Autodesk Fusion 360 part; units mm, degrees
note: some values were not read from the file. Set by a fixed rule: which sketch regions a step uses.
(part 6 of 10)
  spline S32 degree 5 poles (0.6796, -14.5069) (0.6796, -14.507) (0.6797, -14.5072) (0.6797, -14.5074) (0.6797, -14.5078) (0.6797, -14.5083) (0.6798, -14.5089) (0.6798, -14.5096) (0.6799, -14.5104) (0.6799, -14.5112) (0.68, -14.5122) (0.6801, -14.5132) (0.6802, -14.5143) (0.6803, -14.5154) (0.6804, -14.5167) (0.6805, -14.518) (0.6806, -14.5193) (0.6807, -14.5208) (0.6809, -14.5223) (0.681, -14.5239) (0.6812, -14.5256) (0.6814, -14.5273) (0.6815, -14.5291) (0.6817, -14.531) (0.6819, -14.5329) (0.6822, -14.5349) (0.6824, -14.537) (0.6826, -14.5392) (0.6829, -14.5414) (0.6832, -14.5436) (0.6834, -14.546) (0.6837, -14.5484) (0.684, -14.5508) (0.6844, -14.5533) (0.6847, -14.5559) (0.685, -14.5586) (0.6854, -14.5613) (0.6858, -14.5641) (0.6862, -14.5669) (0.6866, -14.5698) (0.687, -14.5727) (0.6874, -14.5757) (0.6879, -14.5788) (0.6883, -14.5819) (0.6888, -14.5851) (0.6893, -14.5883) (0.6898, -14.5916) (0.6904, -14.595) (0.6909, -14.5984) (0.6915, -14.6018) (0.6921, -14.6054) (0.6926, -14.6089) (0.6933, -14.6125) (0.6939, -14.6162) (0.6945, -14.6199) (0.6952, -14.6237) (0.6959, -14.6275) (0.6966, -14.6314) (0.6973, -14.6354) (0.698, -14.6394) (0.6988, -14.6434) (0.6995, -14.6475) (0.7003, -14.6516) (0.7011, -14.6558) (0.702, -14.66) (0.7028, -14.6643) (0.7037, -14.6686) (0.7045, -14.673) (0.7054, -14.6774) (0.7064, -14.6819) (0.7073, -14.6864) (0.7082, -14.691) (0.7092, -14.6956) (0.7102, -14.7003) (0.7112, -14.705) (0.7123, -14.7097) (0.7133, -14.7145) (0.7144, -14.7194) (0.7155, -14.7243) (0.7166, -14.7292) (0.7177, -14.7342) (0.7189, -14.7392) (0.7201, -14.7442) (0.7213, -14.7493) (0.7225, -14.7545) (0.7237, -14.7597) (0.725, -14.7649) (0.7263, -14.7702) (0.7276, -14.7755) (0.7289, -14.7808) (0.7302, -14.7862) (0.7316, -14.7917) (0.733, -14.7971) (0.7344, -14.8027) (0.7358, -14.8082) (0.7372, -14.8138) (0.7387, -14.8194) (0.7402, -14.8251) (0.7417, -14.8308) (0.7433, -14.8366) (0.7448, -14.8424) (0.7464, -14.8482) (0.748, -14.854) (0.7496, -14.86) (0.7513, -14.8659) (0.7529, -14.8719) (0.7546, -14.8779) (0.7564, -14.8839) (0.7581, -14.89) (0.7599, -14.8961) (0.7616, -14.9023) (0.7634, -14.9085) (0.7653, -14.9147) (0.7671, -14.921) (0.769, -14.9273) (0.7709, -14.9336) (0.7728, -14.94) (0.7748, -14.9464) (0.7767, -14.9528) (0.7787, -14.9593) (0.7807, -14.9658) (0.7828, -14.9723) (0.7848, -14.9789) (0.7869, -14.9855) (0.789, -14.9921) (0.7912, -14.9987) (0.7933, -15.0054) (0.7955, -15.0122) (0.7977, -15.0189) (0.8, -15.0257) (0.8022, -15.0325) (0.8045, -15.0394) (0.8068, -15.0463) (0.8091, -15.0532) (0.8115, -15.0601) (0.8138, -15.0671) (0.8162, -15.0741) (0.8187, -15.0812) (0.8211, -15.0882) (0.8236, -15.0953) (0.8261, -15.1025) (0.8286, -15.1096) (0.8311, -15.1168) (0.8337, -15.124) (0.8363, -15.1313) (0.8389, -15.1385) (0.8416, -15.1458) (0.8442, -15.1531) (0.8469, -15.1605) (0.8497, -15.1679) (0.8524, -15.1753) (0.8552, -15.1827) (0.858, -15.1902) (0.8608, -15.1977) (0.8636, -15.2052) (0.8665, -15.2127) (0.8694, -15.2203) (0.8723, -15.2279) (0.8753, -15.2355) (0.8782, -15.2432) (0.8812, -15.2509) (0.8843, -15.2586) (0.8873, -15.2663) (0.8904, -15.274) (0.8935, -15.2818) (0.8966, -15.2896) (0.8998, -15.2974) (0.9029, -15.3053) (0.9061, -15.3132) (0.9094, -15.3211) (0.9126, -15.329) (0.9159, -15.3369) (0.9192, -15.3449) (0.9225, -15.3529) (0.9259, -15.3609) (0.9293, -15.369) (0.9327, -15.377) (0.9361, -15.3851) (0.9396, -15.3932) (0.9431, -15.4014) (0.9466, -15.4095) (0.9501, -15.4177) (0.9537, -15.4259) (0.9573, -15.4341) (0.9609, -15.4424) (0.9646, -15.4507) (0.9682, -15.459) (0.9719, -15.4673) (0.9757, -15.4756) (0.9794, -15.484) (0.9832, -15.4923) (0.987, -15.5007) (0.9908, -15.5091) (0.9947, -15.5176) (0.9986, -15.526) (1.0025, -15.5345) (1.0064, -15.543) (1.0104, -15.5515) (1.0144, -15.5601) (1.0184, -15.5686) (1.0224, -15.5772) (1.0265, -15.5858) (1.0306, -15.5944) (1.0347, -15.6031) (1.0389, -15.6117) (1.043, -15.6204) (1.0472, -15.6291) (1.0515, -15.6378) (1.0557, -15.6466) (1.06, -15.6553) (1.0643, -15.6641) (1.0687, -15.6729) (1.073, -15.6817) (1.0774, -15.6905) (1.0818, -15.6993) (1.0863, -15.7082) (1.0907, -15.7171) (1.0952, -15.726) (1.0998, -15.7349) (1.1043, -15.7438) (1.1089, -15.7528) (1.1135, -15.7617) (1.1182, -15.7707) (1.1228, -15.7797) (1.1275, -15.7887) (1.1322, -15.7977) (1.137, -15.8068) (1.1417, -15.8159) (1.1465, -15.8249) (1.1514, -15.834) (1.1562, -15.8431) (1.1611, -15.8523) (1.166, -15.8614) (1.1709, -15.8706) (1.1759, -15.8797) (1.1809, -15.8889) (1.1859, -15.8981) (1.1909, -15.9074) (1.196, -15.9166) (1.2011, -15.9258) (1.2062, -15.9351) (1.2104, -15.9425) (1.2135, -15.9481) (1.2155, -15.9518) (1.2166, -15.9537) knots 0 0 0 0 0 0 0.00416667 0.00833333 0.0125 0.01666667 0.02083333 0.025 0.02916667 0.03333333 0.0375 0.04166667 0.04583333 0.05 0.05416667 0.05833333 0.0625 0.06666667 0.07083333 0.075 0.07916667 0.08333333 0.0875 0.09166667 0.09583333 0.1 0.10416667 0.10833333 0.1125 0.11666667 0.12083333 0.125 0.12916667 0.13333333 0.1375 0.14166667 0.14583333 0.15 0.15416667 0.15833333 0.1625 0.16666667 0.17083333 0.175 0.17916667 0.18333333 0.1875 0.19166667 0.19583333 0.2 0.20416667 0.20833333 0.2125 0.21666667 0.22083333 0.225 0.22916667 0.23333333 0.2375 0.24166667 0.24583333 0.25 0.25416667 0.25833333 0.2625 0.26666667 0.27083333 0.275 0.27916667 0.28333333 0.2875 0.29166667 0.29583333 0.3 0.30416667 0.30833333 0.3125 0.31666667 0.32083333 0.325 0.32916667 0.33333333 0.3375 0.34166667 0.34583333 0.35 0.35416667 0.35833333 0.3625 0.36666667 0.37083333 0.375 0.37916667 0.38333333 0.3875 0.39166667 0.39583333 0.4 0.40416667 0.40833333 0.4125 0.41666667 0.42083333 0.425 0.42916667 0.43333333 0.4375 0.44166667 0.44583333 0.45 0.45416667 0.45833333 0.4625 0.46666667 0.47083333 0.475 0.47916667 0.48333333 0.4875 0.49166667 0.49583333 0.5 0.50416667 0.50833333 0.5125 0.51666667 0.52083333 0.525 0.52916667 0.53333333 0.5375 0.54166667 0.54583333 0.55 0.55416667 0.55833333 0.5625 0.56666667 0.57083333 0.575 0.57916667 0.58333333 0.5875 0.59166667 0.59583333 0.6 0.60416667 0.60833333 0.6125 0.61666667 0.62083333 0.625 0.62916667 0.63333333 0.6375 0.64166667 0.64583333 0.65 0.65416667 0.65833333 0.6625 0.66666667 0.67083333 0.675 0.67916667 0.68333333 0.6875 0.69166667 0.69583333 0.7 0.70416667 0.70833333 0.7125 0.71666667 0.72083333 0.725 0.72916667 0.73333333 0.7375 0.74166667 0.74583333 0.75 0.75416667 0.75833333 0.7625 0.76666667 0.77083333 0.775 0.77916667 0.78333333 0.7875 0.79166667 0.79583333 0.8 0.80416667 0.80833333 0.8125 0.81666667 0.82083333 0.825 0.82916667 0.83333333 0.8375 0.84166667 0.84583333 0.85 0.85416667 0.85833333 0.8625 0.86666667 0.87083333 0.875 0.87916667 0.88333333 0.8875 0.89166667 0.89583333 0.9 0.90416667 0.90833333 0.9125 0.91666667 0.92083333 0.925 0.92916667 0.93333333 0.9375 0.94166667 0.94583333 0.95 0.95416667 0.95833333 0.9625 0.96666667 0.97083333 0.975 0.97916667 0.98333333 0.9875 0.99166667 0.99583333 1 1 1 1 1 1
  arc A41 (4.5069, -15.3521) -> (5.3776, -15.0692) centre (0, 0) ccw
  spline S33 degree 5 poles (-15.5488, -3.7729) (-15.5467, -3.7733) (-15.5425, -3.7742) (-15.5363, -3.7754) (-15.5279, -3.777) (-15.5175, -3.779) (-15.5072, -3.781) (-15.4968, -3.783) (-15.4865, -3.7849) (-15.4762, -3.7869) (-15.4659, -3.7888) (-15.4556, -3.7907) (-15.4454, -3.7925) (-15.4352, -3.7944) (-15.425, -3.7962) (-15.4148, -3.798) (-15.4047, -3.7998) (-15.3946, -3.8015) (-15.3845, -3.8033) (-15.3744, -3.805) (-15.3644, -3.8067) (-15.3544, -3.8083) (-15.3444, -3.81) (-15.3344, -3.8116) (-15.3244, -3.8132) (-15.3145, -3.8148) (-15.3046, -3.8164) (-15.2947, -3.8179) (-15.2849, -3.8195) (-15.2751, -3.821) (-15.2653, -3.8225) (-15.2555, -3.8239) (-15.2457, -3.8254) (-15.236, -3.8268) (-15.2263, -3.8282) (-15.2166, -3.8296) (-15.207, -3.831) (-15.1974, -3.8323) (-15.1878, -3.8337) (-15.1782, -3.835) (-15.1687, -3.8363) (-15.1591, -3.8375) (-15.1497, -3.8388) (-15.1402, -3.84) (-15.1308, -3.8412) (-15.1214, -3.8424) (-15.112, -3.8436) (-15.1026, -3.8448) (-15.0933, -3.8459) (-15.084, -3.847) (-15.0747, -3.8481) (-15.0655, -3.8492) (-15.0563, -3.8503) (-15.0471, -3.8513) (-15.0379, -3.8523) (-15.0288, -3.8533) (-15.0197, -3.8543) (-15.0106, -3.8553) (-15.0015, -3.8562) (-14.9925, -3.8572) (-14.9835, -3.8581) (-14.9746, -3.859) (-14.9656, -3.8598) (-14.9567, -3.8607) (-14.9479, -3.8615) (-14.939, -3.8624) (-14.9302, -3.8632) (-14.9214, -3.8639) (-14.9127, -3.8647) (-14.9039, -3.8655) (-14.8952, -3.8662) (-14.8866, -3.8669) (-14.8779, -3.8676) (-14.8693, -3.8683) (-14.8608, -3.869) (-14.8522, -3.8696) (-14.8437, -3.8702) (-14.8352, -3.8708) (-14.8268, -3.8714) (-14.8184, -3.872) (-14.81, -3.8726) (-14.8016, -3.8731) (-14.7933, -3.8737) (-14.785, -3.8742) (-14.7768, -3.8747) (-14.7685, -3.8751) (-14.7603, -3.8756) (-14.7522, -3.8761) (-14.744, -3.8765) (-14.7359, -3.8769) (-14.7279, -3.8773) (-14.7199, -3.8777) (-14.7119, -3.878) (-14.7039, -3.8784) (-14.696, -3.8787) (-14.6881, -3.8791) (-14.6802, -3.8794) (-14.6724, -3.8797) (-14.6646, -3.8799) (-14.6568, -3.8802) (-14.6491, -3.8804) (-14.6414, -3.8807) (-14.6338, -3.8809) (-14.6261, -3.8811) (-14.6186, -3.8813) (-14.611, -3.8814) (-14.6035, -3.8816) (-14.596, -3.8817) (-14.5886, -3.8819) (-14.5812, -3.882) (-14.5738, -3.8821) (-14.5665, -3.8822) (-14.5592, -3.8823) (-14.5519, -3.8823) (-14.5447, -3.8824) (-14.5375, -3.8824) (-14.5304, -3.8824) (-14.5233, -3.8824) (-14.5162, -3.8824) (-14.5091, -3.8824) (-14.5021, -3.8824) (-14.4952, -3.8823) (-14.4883, -3.8823) (-14.4814, -3.8822) (-14.4745, -3.8821) (-14.4677, -3.882) (-14.461, -3.8819) (-14.4542, -3.8818) (-14.4476, -3.8817) (-14.4409, -3.8816) (-14.4343, -3.8814) (-14.4277, -3.8812) (-14.4212, -3.8811) (-14.4147, -3.8809) (-14.4083, -3.8807) (-14.4019, -3.8805) (-14.3955, -3.8803) (-14.3892, -3.88) (-14.3829, -3.8798) (-14.3767, -3.8796) (-14.3705, -3.8793) (-14.3643, -3.879) (-14.3582, -3.8788) (-14.3521, -3.8785) (-14.3461, -3.8782) (-14.3401, -3.8779) (-14.3342, -3.8776) (-14.3283, -3.8772) (-14.3224, -3.8769) (-14.3166, -3.8766) (-14.3108, -3.8762) (-14.3051, -3.8758) (-14.2994, -3.8755) (-14.2938, -3.8751) (-14.2882, -3.8747) (-14.2826, -3.8743) (-14.2771, -3.8739) (-14.2717, -3.8735) (-14.2663, -3.8731) (-14.2609, -3.8727) (-14.2556, -3.8723) (-14.2503, -3.8718) (-14.2451, -3.8714) (-14.2399, -3.871) (-14.2348, -3.8705) (-14.2297, -3.87) (-14.2247, -3.8696) (-14.2197, -3.8691) (-14.2148, -3.8686) (-14.2099, -3.8682) (-14.2051, -3.8677) (-14.2003, -3.8672) (-14.1955, -3.8667) (-14.1908, -3.8662) (-14.1862, -3.8657) (-14.1816, -3.8652) (-14.1771, -3.8647) (-14.1726, -3.8642) (-14.1682, -3.8636) (-14.1638, -3.8631) (-14.1594, -3.8626) (-14.1552, -3.8621) (-14.1509, -3.8615) (-14.1467, -3.861) (-14.1426, -3.8605) (-14.1386, -3.86) (-14.1345, -3.8594) (-14.1306, -3.8589) (-14.1267, -3.8583) (-14.1228, -3.8578) (-14.119, -3.8573) (-14.1153, -3.8567) (-14.1116, -3.8562) (-14.1079, -3.8557) (-14.1044, -3.8551) (-14.1009, -3.8546) (-14.0974, -3.854) (-14.094, -3.8535) (-14.0906, -3.853) (-14.0873, -3.8525) (-14.0841, -3.8519) (-14.0809, -3.8514) (-14.0778, -3.8509) (-14.0748, -3.8504) (-14.0718, -3.8498) (-14.0688, -3.8493) (-14.066, -3.8488) (-14.0632, -3.8483) (-14.0604, -3.8478) (-14.0577, -3.8473) (-14.0551, -3.8469) (-14.0525, -3.8464) (-14.05, -3.8459) (-14.0476, -3.8454) (-14.0452, -3.845) (-14.0429, -3.8445) (-14.0407, -3.8441) (-14.0385, -3.8436) (-14.0364, -3.8432) (-14.0343, -3.8428) (-14.0324, -3.8424) (-14.0305, -3.842) (-14.0286, -3.8416) (-14.0268, -3.8412) (-14.0251, -3.8408) (-14.0235, -3.8405) (-14.0219, -3.8401) (-14.0204, -3.8398) (-14.019, -3.8394) (-14.0177, -3.8391) (-14.0164, -3.8388) (-14.0152, -3.8386) (-14.0141, -3.8383) (-14.013, -3.838) (-14.012, -3.8378) (-14.0111, -3.8376) (-14.0103, -3.8374) (-14.0095, -3.8372) (-14.0089, -3.837) (-14.0083, -3.8369) (-14.0077, -3.8367) (-14.0074, -3.8366) (-14.0072, -3.8366) (-14.007, -3.8365) (-14.007, -3.8365) knots -1 -1 -1 -1 -1 -1 -0.99583333 -0.99166667 -0.9875 -0.98333333 -0.97916667 -0.975 -0.97083333 -0.96666667 -0.9625 -0.95833333 -0.95416667 -0.95 -0.94583333 -0.94166667 -0.9375 -0.93333333 -0.92916667 -0.925 -0.92083333 -0.91666667 -0.9125 -0.90833333 -0.90416667 -0.9 -0.89583333 -0.89166667 -0.8875 -0.88333333 -0.87916667 -0.875 -0.87083333 -0.86666667 -0.8625 -0.85833333 -0.85416667 -0.85 -0.84583333 -0.84166667 -0.8375 -0.83333333 -0.82916667 -0.825 -0.82083333 -0.81666667 -0.8125 -0.80833333 -0.80416667 -0.8 -0.79583333 -0.79166667 -0.7875 -0.78333333 -0.77916667 -0.775 -0.77083333 -0.76666667 -0.7625 -0.75833333 -0.75416667 -0.75 -0.74583333 -0.74166667 -0.7375 -0.73333333 -0.72916667 -0.725 -0.72083333 -0.71666667 -0.7125 -0.70833333 -0.70416667 -0.7 -0.69583333 -0.69166667 -0.6875 -0.68333333 -0.67916667 -0.675 -0.67083333 -0.66666667 -0.6625 -0.65833333 -0.65416667 -0.65 -0.64583333 -0.64166667 -0.6375 -0.63333333 -0.62916667 -0.625 -0.62083333 -0.61666667 -0.6125 -0.60833333 -0.60416667 -0.6 -0.59583333 -0.59166667 -0.5875 -0.58333333 -0.57916667 -0.575 -0.57083333 -0.56666667 -0.5625 -0.55833333 -0.55416667 -0.55 -0.54583333 -0.54166667 -0.5375 -0.53333333 -0.52916667 -0.525 -0.52083333 -0.51666667 -0.5125 -0.50833333 -0.50416667 -0.5 -0.49583333 -0.49166667 -0.4875 -0.48333333 -0.47916667 -0.475 -0.47083333 -0.46666667 -0.4625 -0.45833333 -0.45416667 -0.45 -0.44583333 -0.44166667 -0.4375 -0.43333333 -0.42916667 -0.425 -0.42083333 -0.41666667 -0.4125 -0.40833333 -0.40416667 -0.4 -0.39583333 -0.39166667 -0.3875 -0.38333333 -0.37916667 -0.375 -0.37083333 -0.36666667 -0.3625 -0.35833333 -0.35416667 -0.35 -0.34583333 -0.34166667 -0.3375 -0.33333333 -0.32916667 -0.325 -0.32083333 -0.31666667 -0.3125 -0.30833333 -0.30416667 -0.3 -0.29583333 -0.29166667 -0.2875 -0.28333333 -0.27916667 -0.275 -0.27083333 -0.26666667 -0.2625 -0.25833333 -0.25416667 -0.25 -0.24583333 -0.24166667 -0.2375 -0.23333333 -0.22916667 -0.225 -0.22083333 -0.21666667 -0.2125 -0.20833333 -0.20416667 -0.2 -0.19583333 -0.19166667 -0.1875 -0.18333333 -0.17916667 -0.175 -0.17083333 -0.16666667 -0.1625 -0.15833333 -0.15416667 -0.15 -0.14583333 -0.14166667 -0.1375 -0.13333333 -0.12916667 -0.125 -0.12083333 -0.11666667 -0.1125 -0.10833333 -0.10416667 -0.1 -0.09583333 -0.09166667 -0.0875 -0.08333333 -0.07916667 -0.075 -0.07083333 -0.06666667 -0.0625 -0.05833333 -0.05416667 -0.05 -0.04583333 -0.04166667 -0.0375 -0.03333333 -0.02916667 -0.025 -0.02083333 -0.01666667 -0.0125 -0.00833333 -0.00416667 0 0 0 0 0 0
  spline S34 degree 5 poles (-5.3776, 15.0692) (-5.3777, 15.0671) (-5.3781, 15.0629) (-5.3787, 15.0565) (-5.3794, 15.0481) (-5.3804, 15.0375) (-5.3813, 15.027) (-5.3821, 15.0165) (-5.383, 15.006) (-5.3838, 14.9956) (-5.3846, 14.9851) (-5.3854, 14.9747) (-5.3862, 14.9644) (-5.387, 14.954) (-5.3877, 14.9437) (-5.3885, 14.9334) (-5.3892, 14.9231) (-5.3899, 14.9129) (-5.3905, 14.9027) (-5.3912, 14.8925) (-5.3918, 14.8823) (-5.3924, 14.8722) (-5.393, 14.862) (-5.3936, 14.852) (-5.3942, 14.8419) (-5.3947, 14.8319) (-5.3953, 14.8218) (-5.3958, 14.8119) (-5.3963, 14.8019) (-5.3967, 14.792) (-5.3972, 14.7821) (-5.3976, 14.7722) (-5.3981, 14.7624) (-5.3985, 14.7525) (-5.3988, 14.7427) (-5.3992, 14.733) (-5.3996, 14.7232) (-5.3999, 14.7135) (-5.4002, 14.7038) (-5.4005, 14.6942) (-5.4008, 14.6846) (-5.4011, 14.675) (-5.4013, 14.6654) (-5.4016, 14.6559) (-5.4018, 14.6464) (-5.402, 14.6369) (-5.4022, 14.6274) (-5.4024, 14.618) (-5.4025, 14.6086) (-5.4027, 14.5992) (-5.4028, 14.5899) (-5.4029, 14.5806) (-5.403, 14.5713) (-5.4031, 14.5621) (-5.4031, 14.5528) (-5.4032, 14.5437) (-5.4032, 14.5345) (-5.4032, 14.5254) (-5.4032, 14.5163) (-5.4032, 14.5072) (-5.4031, 14.4982) (-5.4031, 14.4892) (-5.403, 14.4802) (-5.403, 14.4712) (-5.4029, 14.4623) (-5.4028, 14.4535) (-5.4026, 14.4446) (-5.4025, 14.4358) (-5.4023, 14.427) (-5.4022, 14.4182) (-5.402, 14.4095) (-5.4018, 14.4008) (-5.4016, 14.3922) (-5.4014, 14.3835) (-5.4011, 14.3749) (-5.4009, 14.3664) (-5.4006, 14.3578) (-5.4003, 14.3493) (-5.4001, 14.3409) (-5.3998, 14.3325) (-5.3994, 14.3241) (-5.3991, 14.3157) (-5.3988, 14.3074) (-5.3984, 14.2991) (-5.398, 14.2908) (-5.3976, 14.2826) (-5.3973, 14.2744) (-5.3968, 14.2662) (-5.3964, 14.2581) (-5.396, 14.25) (-5.3955, 14.2419) (-5.3951, 14.2339) (-5.3946, 14.2259) (-5.3941, 14.2179) (-5.3936, 14.21) (-5.3931, 14.2021) (-5.3926, 14.1943) (-5.3921, 14.1865) (-5.3915, 14.1787) (-5.391, 14.171) (-5.3904, 14.1632) (-5.3899, 14.1556) (-5.3893, 14.1479) (-5.3887, 14.1403) (-5.3881, 14.1328) (-5.3874, 14.1253) (-5.3868, 14.1178) (-5.3862, 14.1103) (-5.3855, 14.1029) (-5.3849, 14.0955) (-5.3842, 14.0882) (-5.3835, 14.0809) (-5.3828, 14.0736) (-5.3821, 14.0664) (-5.3814, 14.0592) (-5.3807, 14.0521) (-5.38, 14.0449) (-5.3793, 14.0379) (-5.3785, 14.0308) (-5.3778, 14.0238) (-5.377, 14.0169) (-5.3762, 14.01) (-5.3755, 14.0031) (-5.3747, 13.9963) (-5.3739, 13.9895) (-5.3731, 13.9827) (-5.3723, 13.976) (-5.3714, 13.9693) (-5.3706, 13.9627) (-5.3698, 13.9561) (-5.3689, 13.9495) (-5.3681, 13.943) (-5.3672, 13.9365) (-5.3664, 13.9301) (-5.3655, 13.9237) (-5.3646, 13.9173) (-5.3638, 13.911) (-5.3629, 13.9048) (-5.362, 13.8986) (-5.3611, 13.8924) (-5.3602, 13.8862) (-5.3593, 13.8801) (-5.3583, 13.8741) (-5.3574, 13.8681) (-5.3565, 13.8621) (-5.3556, 13.8562) (-5.3546, 13.8503) (-5.3537, 13.8445) (-5.3528, 13.8387) (-5.3518, 13.833) (-5.3509, 13.8273) (-5.3499, 13.8216) (-5.3489, 13.816) (-5.348, 13.8104) (-5.347, 13.8049) (-5.3461, 13.7994) (-5.3451, 13.794) (-5.3441, 13.7886) (-5.3431, 13.7833) (-5.3422, 13.778) (-5.3412, 13.7728) (-5.3402, 13.7676) (-5.3392, 13.7624) (-5.3382, 13.7573) (-5.3372, 13.7523) (-5.3363, 13.7473) (-5.3353, 13.7423) (-5.3343, 13.7374) (-5.3333, 13.7325) (-5.3323, 13.7277) (-5.3313, 13.723) (-5.3303, 13.7183) (-5.3293, 13.7136) (-5.3284, 13.709) (-5.3274, 13.7044) (-5.3264, 13.6999) (-5.3254, 13.6954) (-5.3244, 13.691) (-5.3235, 13.6867) (-5.3225, 13.6824) (-5.3215, 13.6781) (-5.3205, 13.6739) (-5.3196, 13.6698) (-5.3186, 13.6657) (-5.3176, 13.6616) (-5.3167, 13.6576) (-5.3157, 13.6537) (-5.3148, 13.6498) (-5.3138, 13.646) (-5.3129, 13.6422) (-5.312, 13.6385) (-5.3111, 13.6348) (-5.3101, 13.6312) (-5.3092, 13.6276) (-5.3083, 13.6241) (-5.3074, 13.6207) (-5.3065, 13.6173) (-5.3056, 13.614) (-5.3047, 13.6107) (-5.3039, 13.6075) (-5.303, 13.6043) (-5.3022, 13.6012) (-5.3013, 13.5982) (-5.3005, 13.5952) (-5.2997, 13.5923) (-5.2988, 13.5894) (-5.298, 13.5866) (-5.2972, 13.5839) (-5.2965, 13.5812) (-5.2957, 13.5786) (-5.2949, 13.576) (-5.2942, 13.5735) (-5.2935, 13.5711) (-5.2927, 13.5687) (-5.292, 13.5664) (-5.2913, 13.5641) (-5.2907, 13.5619) (-5.29, 13.5598) (-5.2893, 13.5578) (-5.2887, 13.5558) (-5.2881, 13.5539) (-5.2875, 13.552) (-5.2869, 13.5502) (-5.2863, 13.5485) (-5.2858, 13.5468) (-5.2853, 13.5452) (-5.2848, 13.5437) (-5.2843, 13.5423) (-5.2838, 13.5409) (-5.2833, 13.5396) (-5.2829, 13.5383) (-5.2825, 13.5372) (-5.2821, 13.5361) (-5.2818, 13.5351) (-5.2814, 13.5341) (-5.2811, 13.5332) (-5.2808, 13.5324) (-5.2805, 13.5317) (-5.2803, 13.531) (-5.2801, 13.5305) (-5.2799, 13.53) (-5.2798, 13.5296) (-5.2797, 13.5294) (-5.2796, 13.5293) (-5.2796, 13.5292) knots -1 -1 -1 -1 -1 -1 -0.99583333 -0.99166667 -0.9875 -0.98333333 -0.97916667 -0.975 -0.97083333 -0.96666667 -0.9625 -0.95833333 -0.95416667 -0.95 -0.94583333 -0.94166667 -0.9375 -0.93333333 -0.92916667 -0.925 -0.92083333 -0.91666667 -0.9125 -0.90833333 -0.90416667 -0.9 -0.89583333 -0.89166667 -0.8875 -0.88333333 -0.87916667 -0.875 -0.87083333 -0.86666667 -0.8625 -0.85833333 -0.85416667 -0.85 -0.84583333 -0.84166667 -0.8375 -0.83333333 -0.82916667 -0.825 -0.82083333 -0.81666667 -0.8125 -0.80833333 -0.80416667 -0.8 -0.79583333 -0.79166667 -0.7875 -0.78333333 -0.77916667 -0.775 -0.77083333 -0.76666667 -0.7625 -0.75833333 -0.75416667 -0.75 -0.74583333 -0.74166667 -0.7375 -0.73333333 -0.72916667 -0.725 -0.72083333 -0.71666667 -0.7125 -0.70833333 -0.70416667 -0.7 -0.69583333 -0.69166667 -0.6875 -0.68333333 -0.67916667 -0.675 -0.67083333 -0.66666667 -0.6625 -0.65833333 -0.65416667 -0.65 -0.64583333 -0.64166667 -0.6375 -0.63333333 -0.62916667 -0.625 -0.62083333 -0.61666667 -0.6125 -0.60833333 -0.60416667 -0.6 -0.59583333 -0.59166667 -0.5875 -0.58333333 -0.57916667 -0.575 -0.57083333 -0.56666667 -0.5625 -0.55833333 -0.55416667 -0.55 -0.54583333 -0.54166667 -0.5375 -0.53333333 -0.52916667 -0.525 -0.52083333 -0.51666667 -0.5125 -0.50833333 -0.50416667 -0.5 -0.49583333 -0.49166667 -0.4875 -0.48333333 -0.47916667 -0.475 -0.47083333 -0.46666667 -0.4625 -0.45833333 -0.45416667 -0.45 -0.44583333 -0.44166667 -0.4375 -0.43333333 -0.42916667 -0.425 -0.42083333 -0.41666667 -0.4125 -0.40833333 -0.40416667 -0.4 -0.39583333 -0.39166667 -0.3875 -0.38333333 -0.37916667 -0.375 -0.37083333 -0.36666667 -0.3625 -0.35833333 -0.35416667 -0.35 -0.34583333 -0.34166667 -0.3375 -0.33333333 -0.32916667 -0.325 -0.32083333 -0.31666667 -0.3125 -0.30833333 -0.30416667 -0.3 -0.29583333 -0.29166667 -0.2875 -0.28333333 -0.27916667 -0.275 -0.27083333 -0.26666667 -0.2625 -0.25833333 -0.25416667 -0.25 -0.24583333 -0.24166667 -0.2375 -0.23333333 -0.22916667 -0.225 -0.22083333 -0.21666667 -0.2125 -0.20833333 -0.20416667 -0.2 -0.19583333 -0.19166667 -0.1875 -0.18333333 -0.17916667 -0.175 -0.17083333 -0.16666667 -0.1625 -0.15833333 -0.15416667 -0.15 -0.14583333 -0.14166667 -0.1375 -0.13333333 -0.12916667 -0.125 -0.12083333 -0.11666667 -0.1125 -0.10833333 -0.10416667 -0.1 -0.09583333 -0.09166667 -0.0875 -0.08333333 -0.07916667 -0.075 -0.07083333 -0.06666667 -0.0625 -0.05833333 -0.05416667 -0.05 -0.04583333 -0.04166667 -0.0375 -0.03333333 -0.02916667 -0.025 -0.02083333 -0.01666667 -0.0125 -0.00833333 -0.00416667 0 0 0 0 0 0
  arc A42 (-4.9987, 12.8092) -> (-6.1743, 12.2858) centre (0, 0) ccw
  arc A43 (-2.2262, 13.5686) -> (-3.4851, 13.301) centre (0, 0) ccw
  circle A44 centre (0, 10) radius 1.7
  line L79 (2.3513, 14.3306) -> (2.3514, 14.3312)
  line L80 (-5.2794, 13.5286) -> (-4.9987, 12.8092)
  spline S35 degree 5 poles (-12.6699, -9.771) (-12.6679, -9.7705) (-12.6637, -9.7696) (-12.6575, -9.7682) (-12.6492, -9.7663) (-12.6389, -9.7639) (-12.6286, -9.7615) (-12.6184, -9.7591) (-12.6081, -9.7566) (-12.5979, -9.7542) (-12.5878, -9.7518) (-12.5776, -9.7493) (-12.5675, -9.7469) (-12.5574, -9.7444) (-12.5474, -9.7419) (-12.5374, -9.7394) (-12.5274, -9.7369) (-12.5174, -9.7344) (-12.5075, -9.7319) (-12.4976, -9.7293) (-12.4877, -9.7268) (-12.4779, -9.7243) (-12.4681, -9.7217) (-12.4583, -9.7191) (-12.4486, -9.7166) (-12.4389, -9.714) (-12.4292, -9.7114) (-12.4195, -9.7088) (-12.4099, -9.7062) (-12.4003, -9.7036) (-12.3908, -9.7009) (-12.3812, -9.6983) (-12.3717, -9.6957) (-12.3623, -9.693) (-12.3528, -9.6904) (-12.3434, -9.6877) (-12.3341, -9.685) (-12.3247, -9.6823) (-12.3154, -9.6797) (-12.3062, -9.677) (-12.2969, -9.6743) (-12.2877, -9.6716) (-12.2785, -9.6688) (-12.2694, -9.6661) (-12.2603, -9.6634) (-12.2512, -9.6607) (-12.2421, -9.6579) (-12.2331, -9.6552) (-12.2241, -9.6524) (-12.2152, -9.6496) (-12.2063, -9.6469) (-12.1974, -9.6441) (-12.1885, -9.6413) (-12.1797, -9.6385) (-12.1709, -9.6357) (-12.1622, -9.6329) (-12.1535, -9.6301) (-12.1448, -9.6273) (-12.1361, -9.6245) (-12.1275, -9.6217) (-12.1189, -9.6189) (-12.1104, -9.616) (-12.1018, -9.6132) (-12.0934, -9.6104) (-12.0849, -9.6075) (-12.0765, -9.6047) (-12.0681, -9.6018) (-12.0598, -9.599) (-12.0515, -9.5961) (-12.0432, -9.5933) (-12.035, -9.5904) (-12.0267, -9.5875) (-12.0186, -9.5846) (-12.0104, -9.5818) (-12.0023, -9.5789) (-11.9943, -9.576) (-11.9862, -9.5731) (-11.9782, -9.5702) (-11.9703, -9.5673) (-11.9624, -9.5644) (-11.9545, -9.5615) (-11.9466, -9.5586) (-11.9388, -9.5557) (-11.931, -9.5528) (-11.9233, -9.5499) (-11.9156, -9.547) (-11.9079, -9.5441) (-11.9002, -9.5412) (-11.8926, -9.5383) (-11.8851, -9.5354) (-11.8776, -9.5325) (-11.8701, -9.5295) (-11.8626, -9.5266) (-11.8552, -9.5237) (-11.8478, -9.5208) (-11.8405, -9.5179) (-11.8332, -9.515) (-11.8259, -9.512) (-11.8187, -9.5091) (-11.8115, -9.5062) (-11.8043, -9.5033) (-11.7972, -9.5004) (-11.7901, -9.4975) (-11.7831, -9.4945) (-11.7761, -9.4916) (-11.7691, -9.4887) (-11.7622, -9.4858) (-11.7553, -9.4829) (-11.7484, -9.48) (-11.7416, -9.4771) (-11.7348, -9.4742) (-11.7281, -9.4713) (-11.7214, -9.4684) (-11.7148, -9.4655) (-11.7081, -9.4626) (-11.7016, -9.4597) (-11.695, -9.4568) (-11.6885, -9.4539) (-11.6821, -9.451) (-11.6756, -9.4482) (-11.6693, -9.4453) (-11.6629, -9.4424) (-11.6566, -9.4396) (-11.6504, -9.4367) (-11.6441, -9.4338) (-11.638, -9.431) (-11.6318, -9.4281) (-11.6257, -9.4253) (-11.6197, -9.4225) (-11.6137, -9.4196) (-11.6077, -9.4168) (-11.6017, -9.414) (-11.5959, -9.4112) (-11.59, -9.4084) (-11.5842, -9.4056) (-11.5784, -9.4028) (-11.5727, -9.4) (-11.567, -9.3972) (-11.5614, -9.3944) (-11.5558, -9.3917) (-11.5502, -9.3889) (-11.5447, -9.3862) (-11.5392, -9.3834) (-11.5338, -9.3807) (-11.5284, -9.378) (-11.5231, -9.3753) (-11.5178, -9.3725) (-11.5125, -9.3699) (-11.5073, -9.3672) (-11.5021, -9.3645) (-11.497, -9.3618) (-11.4919, -9.3592) (-11.4869, -9.3565) (-11.4819, -9.3539) (-11.4769, -9.3513) (-11.472, -9.3487) (-11.4672, -9.3461) (-11.4623, -9.3435) (-11.4576, -9.3409) (-11.4528, -9.3383) (-11.4482, -9.3358) (-11.4435, -9.3332) (-11.4389, -9.3307) (-11.4344, -9.3282) (-11.4299, -9.3257) (-11.4254, -9.3232) (-11.421, -9.3207) (-11.4167, -9.3183) (-11.4123, -9.3158) (-11.4081, -9.3134) (-11.4038, -9.311) (-11.3997, -9.3086) (-11.3955, -9.3062) (-11.3915, -9.3039) (-11.3874, -9.3015) (-11.3834, -9.2992) (-11.3795, -9.2969) (-11.3756, -9.2946) (-11.3718, -9.2923) (-11.368, -9.2901) (-11.3642, -9.2878) (-11.3605, -9.2856) (-11.3569, -9.2834) (-11.3533, -9.2812) (-11.3497, -9.2791) (-11.3462, -9.2769) (-11.3428, -9.2748) (-11.3394, -9.2727) (-11.336, -9.2706) (-11.3327, -9.2685) (-11.3295, -9.2665) (-11.3263, -9.2645) (-11.3231, -9.2625) (-11.32, -9.2605) (-11.317, -9.2586) (-11.314, -9.2567) (-11.311, -9.2548) (-11.3081, -9.2529) (-11.3053, -9.2511) (-11.3025, -9.2492) (-11.2998, -9.2474) (-11.2971, -9.2457) (-11.2944, -9.2439) (-11.2919, -9.2422) (-11.2893, -9.2405) (-11.2869, -9.2389) (-11.2844, -9.2372) (-11.2821, -9.2356) (-11.2798, -9.2341) (-11.2775, -9.2325) (-11.2753, -9.231) (-11.2732, -9.2295) (-11.2711, -9.2281) (-11.269, -9.2266) (-11.2671, -9.2253) (-11.2651, -9.2239) (-11.2633, -9.2226) (-11.2615, -9.2213) (-11.2597, -9.22) (-11.258, -9.2188) (-11.2564, -9.2177) (-11.2548, -9.2165) (-11.2533, -9.2154) (-11.2518, -9.2143) (-11.2504, -9.2133) (-11.2491, -9.2123) (-11.2478, -9.2113) (-11.2465, -9.2104) (-11.2454, -9.2096) (-11.2443, -9.2087) (-11.2432, -9.2079) (-11.2422, -9.2072) (-11.2413, -9.2065) (-11.2404, -9.2058) (-11.2396, -9.2052) (-11.2389, -9.2046) (-11.2382, -9.2041) (-11.2376, -9.2036) (-11.2371, -9.2032) (-11.2366, -9.2028) (-11.2362, -9.2025) (-11.2359, -9.2022) (-11.2357, -9.2021) (-11.2356, -9.202) (-11.2355, -9.202) knots -1 -1 -1 -1 -1 -1 -0.99583333 -0.99166667 -0.9875 -0.98333333 -0.97916667 -0.975 -0.97083333 -0.96666667 -0.9625 -0.95833333 -0.95416667 -0.95 -0.94583333 -0.94166667 -0.9375 -0.93333333 -0.92916667 -0.925 -0.92083333 -0.91666667 -0.9125 -0.90833333 -0.90416667 -0.9 -0.89583333 -0.89166667 -0.8875 -0.88333333 -0.87916667 -0.875 -0.87083333 -0.86666667 -0.8625 -0.85833333 -0.85416667 -0.85 -0.84583333 -0.84166667 -0.8375 -0.83333333 -0.82916667 -0.825 -0.82083333 -0.81666667 -0.8125 -0.80833333 -0.80416667 -0.8 -0.79583333 -0.79166667 -0.7875 -0.78333333 -0.77916667 -0.775 -0.77083333 -0.76666667 -0.7625 -0.75833333 -0.75416667 -0.75 -0.74583333 -0.74166667 -0.7375 -0.73333333 -0.72916667 -0.725 -0.72083333 -0.71666667 -0.7125 -0.70833333 -0.70416667 -0.7 -0.69583333 -0.69166667 -0.6875 -0.68333333 -0.67916667 -0.675 -0.67083333 -0.66666667 -0.6625 -0.65833333 -0.65416667 -0.65 -0.64583333 -0.64166667 -0.6375 -0.63333333 -0.62916667 -0.625 -0.62083333 -0.61666667 -0.6125 -0.60833333 -0.60416667 -0.6 -0.59583333 -0.59166667 -0.5875 -0.58333333 -0.57916667 -0.575 -0.57083333 -0.56666667 -0.5625 -0.55833333 -0.55416667 -0.55 -0.54583333 -0.54166667 -0.5375 -0.53333333 -0.52916667 -0.525 -0.52083333 -0.51666667 -0.5125 -0.50833333 -0.50416667 -0.5 -0.49583333 -0.49166667 -0.4875 -0.48333333 -0.47916667 -0.475 -0.47083333 -0.46666667 -0.4625 -0.45833333 -0.45416667 -0.45 -0.44583333 -0.44166667 -0.4375 -0.43333333 -0.42916667 -0.425 -0.42083333 -0.41666667 -0.4125 -0.40833333 -0.40416667 -0.4 -0.39583333 -0.39166667 -0.3875 -0.38333333 -0.37916667 -0.375 -0.37083333 -0.36666667 -0.3625 -0.35833333 -0.35416667 -0.35 -0.34583333 -0.34166667 -0.3375 -0.33333333 -0.32916667 -0.325 -0.32083333 -0.31666667 -0.3125 -0.30833333 -0.30416667 -0.3 -0.29583333 -0.29166667 -0.2875 -0.28333333 -0.27916667 -0.275 -0.27083333 -0.26666667 -0.2625 -0.25833333 -0.25416667 -0.25 -0.24583333 -0.24166667 -0.2375 -0.23333333 -0.22916667 -0.225 -0.22083333 -0.21666667 -0.2125 -0.20833333 -0.20416667 -0.2 -0.19583333 -0.19166667 -0.1875 -0.18333333 -0.17916667 -0.175 -0.17083333 -0.16666667 -0.1625 -0.15833333 -0.15416667 -0.15 -0.14583333 -0.14166667 -0.1375 -0.13333333 -0.12916667 -0.125 -0.12083333 -0.11666667 -0.1125 -0.10833333 -0.10416667 -0.1 -0.09583333 -0.09166667 -0.0875 -0.08333333 -0.07916667 -0.075 -0.07083333 -0.06666667 -0.0625 -0.05833333 -0.05416667 -0.05 -0.04583333 -0.04166667 -0.0375 -0.03333333 -0.02916667 -0.025 -0.02083333 -0.01666667 -0.0125 -0.00833333 -0.00416667 0 0 0 0 0 0
  spline S36 degree 5 poles (-12.9032, 6.6649) (-12.9033, 6.6649) (-12.9034, 6.665) (-12.9036, 6.6651) (-12.9039, 6.6652) (-12.9044, 6.6655) (-12.905, 6.6658) (-12.9056, 6.6661) (-12.9063, 6.6664) (-12.9071, 6.6668) (-12.9079, 6.6672) (-12.9088, 6.6676) (-12.9098, 6.6681) (-12.9108, 6.6686) (-12.912, 6.6691) (-12.9132, 6.6697) (-12.9144, 6.6703) (-12.9157, 6.6709) (-12.9171, 6.6715) (-12.9186, 6.6722) (-12.9201, 6.6729) (-12.9217, 6.6736) (-12.9234, 6.6743) (-12.9251, 6.6751) (-12.9269, 6.6759) (-12.9287, 6.6767) (-12.9306, 6.6775) (-12.9326, 6.6784) (-12.9346, 6.6793) (-12.9367, 6.6802) (-12.9389, 6.6811) (-12.9411, 6.6821) (-12.9434, 6.683) (-12.9457, 6.684) (-12.9482, 6.685) (-12.9506, 6.686) (-12.9531, 6.6871) (-12.9557, 6.6881) (-12.9584, 6.6892) (-12.9611, 6.6903) (-12.9638, 6.6914) (-12.9667, 6.6925) (-12.9695, 6.6937) (-12.9725, 6.6948) (-12.9755, 6.696) (-12.9785, 6.6972) (-12.9816, 6.6984) (-12.9848, 6.6996) (-12.988, 6.7008) (-12.9913, 6.7021) (-12.9946, 6.7033) (-12.998, 6.7046) (-13.0015, 6.7059) (-13.005, 6.7072) (-13.0085, 6.7085) (-13.0121, 6.7098) (-13.0158, 6.7111) (-13.0195, 6.7125) (-13.0232, 6.7138) (-13.0271, 6.7152) (-13.0309, 6.7165) (-13.0349, 6.7179) (-13.0388, 6.7193) (-13.0429, 6.7207) (-13.0469, 6.7221) (-13.0511, 6.7235) (-13.0552, 6.7249) (-13.0595, 6.7264) (-13.0638, 6.7278) (-13.0681, 6.7292) (-13.0725, 6.7307) (-13.0769, 6.7321) (-13.0814, 6.7336) (-13.0859, 6.7351) (-13.0905, 6.7366) (-13.0951, 6.738) (-13.0998, 6.7395) (-13.1046, 6.741) (-13.1093, 6.7425) (-13.1142, 6.744) (-13.119, 6.7455) (-13.124, 6.747) (-13.1289, 6.7485) (-13.1339, 6.75) (-13.139, 6.7516) (-13.1441, 6.7531) (-13.1493, 6.7546) (-13.1545, 6.7561) (-13.1597, 6.7577) (-13.165, 6.7592) (-13.1704, 6.7607) (-13.1758, 6.7623) (-13.1812, 6.7638) (-13.1867, 6.7653) (-13.1922, 6.7669) (-13.1978, 6.7684) (-13.2034, 6.77) (-13.209, 6.7715) (-13.2147, 6.7731) (-13.2205, 6.7746) (-13.2263, 6.7761) (-13.2321, 6.7777) (-13.238, 6.7792) (-13.2439, 6.7808) (-13.2499, 6.7823) (-13.2559, 6.7839) (-13.2619, 6.7854) (-13.268, 6.7869) (-13.2742, 6.7885) (-13.2804, 6.79) (-13.2866, 6.7915) (-13.2928, 6.7931) (-13.2991, 6.7946) (-13.3055, 6.7961) (-13.3119, 6.7976) (-13.3183, 6.7992) (-13.3248, 6.8007) (-13.3313, 6.8022) (-13.3379, 6.8037) (-13.3445, 6.8052) (-13.3511, 6.8067) (-13.3578, 6.8082) (-13.3645, 6.8097) (-13.3712, 6.8112) (-13.378, 6.8127) (-13.3849, 6.8142) (-13.3918, 6.8157) (-13.3987, 6.8171) (-13.4056, 6.8186) (-13.4126, 6.8201) (-13.4197, 6.8215) (-13.4267, 6.823) (-13.4339, 6.8244) (-13.441, 6.8259) (-13.4482, 6.8273) (-13.4554, 6.8288) (-13.4627, 6.8302) (-13.47, 6.8316) (-13.4773, 6.833) (-13.4847, 6.8344) (-13.4922, 6.8358) (-13.4996, 6.8372) (-13.5071, 6.8386) (-13.5146, 6.84) (-13.5222, 6.8414) (-13.5298, 6.8427) (-13.5375, 6.8441) (-13.5451, 6.8454) (-13.5528, 6.8468) (-13.5606, 6.8481) (-13.5684, 6.8494) (-13.5762, 6.8508) (-13.5841, 6.8521) (-13.592, 6.8534) (-13.5999, 6.8547) (-13.6079, 6.856) (-13.6159, 6.8572) (-13.6239, 6.8585) (-13.632, 6.8598) (-13.6401, 6.861) (-13.6483, 6.8623) (-13.6564, 6.8635) (-13.6647, 6.8647) (-13.6729, 6.8659) (-13.6812, 6.8671) (-13.6895, 6.8683) (-13.6979, 6.8695) (-13.7063, 6.8707) (-13.7147, 6.8718) (-13.7231, 6.873) (-13.7316, 6.8741) (-13.7401, 6.8753) (-13.7487, 6.8764) (-13.7573, 6.8775) (-13.7659, 6.8786) (-13.7746, 6.8797) (-13.7833, 6.8808) (-13.792, 6.8818) (-13.8007, 6.8829) (-13.8095, 6.884) (-13.8184, 6.885) (-13.8272, 6.886) (-13.8361, 6.887) (-13.845, 6.888) (-13.854, 6.889) (-13.8629, 6.89) (-13.872, 6.891) (-13.881, 6.8919) (-13.8901, 6.8929) (-13.8992, 6.8938) (-13.9083, 6.8947) (-13.9175, 6.8956) (-13.9267, 6.8965) (-13.936, 6.8974) (-13.9452, 6.8982) (-13.9545, 6.8991) (-13.9639, 6.8999) (-13.9732, 6.9008) (-13.9826, 6.9016) (-13.992, 6.9024) (-14.0015, 6.9032) (-14.011, 6.9039) (-14.0205, 6.9047) (-14.03, 6.9055) (-14.0396, 6.9062) (-14.0492, 6.9069) (-14.0588, 6.9076) (-14.0685, 6.9083) (-14.0782, 6.909) (-14.0879, 6.9097) (-14.0976, 6.9103) (-14.1074, 6.9109) (-14.1172, 6.9116) (-14.1271, 6.9122) (-14.1369, 6.9128) (-14.1468, 6.9134) (-14.1568, 6.9139) (-14.1667, 6.9145) (-14.1767, 6.915) (-14.1867, 6.9155) (-14.1967, 6.916) (-14.2068, 6.9165) (-14.2169, 6.917) (-14.227, 6.9175) (-14.2372, 6.9179) (-14.2474, 6.9183) (-14.2576, 6.9188) (-14.2678, 6.9192) (-14.2781, 6.9195) (-14.2883, 6.9199) (-14.2987, 6.9203) (-14.309, 6.9206) (-14.3194, 6.9209) (-14.3298, 6.9212) (-14.3402, 6.9215) (-14.3507, 6.9218) (-14.3611, 6.9221) (-14.3716, 6.9223) (-14.3822, 6.9225) (-14.3927, 6.9227) (-14.4033, 6.9229) (-14.4118, 6.9231) (-14.4182, 6.9232) (-14.4224, 6.9232) (-14.4246, 6.9233) knots 0 0 0 0 0 0 0.00416667 0.00833333 0.0125 0.01666667 0.02083333 0.025 0.02916667 0.03333333 0.0375 0.04166667 0.04583333 0.05 0.05416667 0.05833333 0.0625 0.06666667 0.07083333 0.075 0.07916667 0.08333333 0.0875 0.09166667 0.09583333 0.1 0.10416667 0.10833333 0.1125 0.11666667 0.12083333 0.125 0.12916667 0.13333333 0.1375 0.14166667 0.14583333 0.15 0.15416667 0.15833333 0.1625 0.16666667 0.17083333 0.175 0.17916667 0.18333333 0.1875 0.19166667 0.19583333 0.2 0.20416667 0.20833333 0.2125 0.21666667 0.22083333 0.225 0.22916667 0.23333333 0.2375 0.24166667 0.24583333 0.25 0.25416667 0.25833333 0.2625 0.26666667 0.27083333 0.275 0.27916667 0.28333333 0.2875 0.29166667 0.29583333 0.3 0.30416667 0.30833333 0.3125 0.31666667 0.32083333 0.325 0.32916667 0.33333333 0.3375 0.34166667 0.34583333 0.35 0.35416667 0.35833333 0.3625 0.36666667 0.37083333 0.375 0.37916667 0.38333333 0.3875 0.39166667 0.39583333 0.4 0.40416667 0.40833333 0.4125 0.41666667 0.42083333 0.425 0.42916667 0.43333333 0.4375 0.44166667 0.44583333 0.45 0.45416667 0.45833333 0.4625 0.46666667 0.47083333 0.475 0.47916667 0.48333333 0.4875 0.49166667 0.49583333 0.5 0.50416667 0.50833333 0.5125 0.51666667 0.52083333 0.525 0.52916667 0.53333333 0.5375 0.54166667 0.54583333 0.55 0.55416667 0.55833333 0.5625 0.56666667 0.57083333 0.575 0.57916667 0.58333333 0.5875 0.59166667 0.59583333 0.6 0.60416667 0.60833333 0.6125 0.61666667 0.62083333 0.625 0.62916667 0.63333333 0.6375 0.64166667 0.64583333 0.65 0.65416667 0.65833333 0.6625 0.66666667 0.67083333 0.675 0.67916667 0.68333333 0.6875 0.69166667 0.69583333 0.7 0.70416667 0.70833333 0.7125 0.71666667 0.72083333 0.725 0.72916667 0.73333333 0.7375 0.74166667 0.74583333 0.75 0.75416667 0.75833333 0.7625 0.76666667 0.77083333 0.775 0.77916667 0.78333333 0.7875 0.79166667 0.79583333 0.8 0.80416667 0.80833333 0.8125 0.81666667 0.82083333 0.825 0.82916667 0.83333333 0.8375 0.84166667 0.84583333 0.85 0.85416667 0.85833333 0.8625 0.86666667 0.87083333 0.875 0.87916667 0.88333333 0.8875 0.89166667 0.89583333 0.9 0.90416667 0.90833333 0.9125 0.91666667 0.92083333 0.925 0.92916667 0.93333333 0.9375 0.94166667 0.94583333 0.95 0.95416667 0.95833333 0.9625 0.96666667 0.97083333 0.975 0.97916667 0.98333333 0.9875 0.99166667 0.99583333 1 1 1 1 1 1
  line L81 (-13.5863, 5.129) -> (-12.8639, 4.8563)
  spline S37 degree 5 poles (-14.7969, 6.087) (-14.7955, 6.0854) (-14.7926, 6.0823) (-14.7882, 6.0776) (-14.7824, 6.0714) (-14.7752, 6.0637) (-14.768, 6.056) (-14.7608, 6.0483) (-14.7536, 6.0406) (-14.7464, 6.033) (-14.7392, 6.0254) (-14.732, 6.0179) (-14.7248, 6.0104) (-14.7176, 6.0029) (-14.7104, 5.9954) (-14.7033, 5.988) (-14.6961, 5.9806) (-14.689, 5.9732) (-14.6818, 5.9659) (-14.6747, 5.9586) (-14.6675, 5.9513) (-14.6604, 5.9441) (-14.6533, 5.9368) (-14.6462, 5.9297) (-14.6391, 5.9225) (-14.632, 5.9154) (-14.6249, 5.9083) (-14.6178, 5.9012) (-14.6108, 5.8942) (-14.6037, 5.8872) (-14.5966, 5.8802) (-14.5896, 5.8733) (-14.5826, 5.8664) (-14.5755, 5.8595) (-14.5685, 5.8527) (-14.5615, 5.8459) (-14.5545, 5.8391) (-14.5475, 5.8324) (-14.5405, 5.8256) (-14.5336, 5.819) (-14.5266, 5.8123) (-14.5197, 5.8057) (-14.5127, 5.7991) (-14.5058, 5.7925) (-14.4989, 5.786) (-14.492, 5.7795) (-14.4851, 5.773) (-14.4782, 5.7666) (-14.4713, 5.7602) (-14.4644, 5.7538) (-14.4576, 5.7475) (-14.4507, 5.7412) (-14.4439, 5.7349) (-14.4371, 5.7287) (-14.4303, 5.7225) (-14.4235, 5.7163) (-14.4167, 5.7101) (-14.4099, 5.704) (-14.4031, 5.6979) (-14.3964, 5.6919) (-14.3896, 5.6859) (-14.3829, 5.6799) (-14.3762, 5.6739) (-14.3695, 5.668) (-14.3628, 5.6621) (-14.3562, 5.6562) (-14.3495, 5.6504) (-14.3429, 5.6446) (-14.3362, 5.6388) (-14.3296, 5.6331) (-14.323, 5.6274) (-14.3164, 5.6217) (-14.3098, 5.6161) (-14.3033, 5.6105) (-14.2967, 5.6049) (-14.2902, 5.5993) (-14.2837, 5.5938) (-14.2772, 5.5883) (-14.2707, 5.5829) (-14.2642, 5.5775) (-14.2578, 5.5721) (-14.2513, 5.5667) (-14.2449, 5.5614) (-14.2385, 5.5561) (-14.2321, 5.5509) (-14.2257, 5.5457) (-14.2194, 5.5405) (-14.213, 5.5353) (-14.2067, 5.5302) (-14.2004, 5.5251) (-14.1941, 5.52) (-14.1879, 5.515) (-14.1816, 5.51) (-14.1754, 5.505) (-14.1692, 5.5001) (-14.163, 5.4952) (-14.1568, 5.4903) (-14.1506, 5.4855) (-14.1445, 5.4807) (-14.1383, 5.4759) (-14.1322, 5.4712) (-14.1262, 5.4665) (-14.1201, 5.4618) (-14.114, 5.4572) (-14.108, 5.4526) (-14.102, 5.448) (-14.096, 5.4434) (-14.0901, 5.4389) (-14.0841, 5.4344) (-14.0782, 5.43) (-14.0723, 5.4256) (-14.0664, 5.4212) (-14.0606, 5.4169) (-14.0547, 5.4125) (-14.0489, 5.4083) (-14.0431, 5.404) (-14.0373, 5.3998) (-14.0316, 5.3956) (-14.0259, 5.3914) (-14.0202, 5.3873) (-14.0145, 5.3832) (-14.0088, 5.3792) (-14.0032, 5.3752) (-13.9976, 5.3712) (-13.992, 5.3672) (-13.9865, 5.3633) (-13.9809, 5.3594) (-13.9754, 5.3555) (-13.9699, 5.3517) (-13.9645, 5.3479) (-13.959, 5.3441) (-13.9536, 5.3404) (-13.9482, 5.3367) (-13.9429, 5.3331) (-13.9376, 5.3294) (-13.9322, 5.3258) (-13.927, 5.3223) (-13.9217, 5.3187) (-13.9165, 5.3152) (-13.9113, 5.3118) (-13.9061, 5.3083) (-13.901, 5.3049) (-13.8959, 5.3015) (-13.8908, 5.2982) (-13.8858, 5.2949) (-13.8807, 5.2916) (-13.8757, 5.2884) (-13.8708, 5.2852) (-13.8658, 5.282) (-13.8609, 5.2789) (-13.8561, 5.2758) (-13.8512, 5.2727) (-13.8464, 5.2697) (-13.8416, 5.2666) (-13.8369, 5.2637) (-13.8322, 5.2607) (-13.8275, 5.2578) (-13.8228, 5.2549) (-13.8182, 5.2521) (-13.8136, 5.2493) (-13.8091, 5.2465) (-13.8046, 5.2438) (-13.8001, 5.241) (-13.7956, 5.2384) (-13.7912, 5.2357) (-13.7869, 5.2331) (-13.7825, 5.2305) (-13.7782, 5.228) (-13.7739, 5.2254) (-13.7697, 5.223) (-13.7655, 5.2205) (-13.7613, 5.2181) (-13.7572, 5.2157) (-13.7531, 5.2134) (-13.7491, 5.211) (-13.7451, 5.2087) (-13.7411, 5.2065) (-13.7372, 5.2043) (-13.7333, 5.2021) (-13.7294, 5.1999) (-13.7256, 5.1978) (-13.7218, 5.1957) (-13.7181, 5.1936) (-13.7144, 5.1916) (-13.7108, 5.1896) (-13.7072, 5.1877) (-13.7036, 5.1857) (-13.7001, 5.1838) (-13.6966, 5.182) (-13.6932, 5.1801) (-13.6898, 5.1783) (-13.6864, 5.1766) (-13.6831, 5.1749) (-13.6799, 5.1732) (-13.6767, 5.1715) (-13.6735, 5.1698) (-13.6704, 5.1682) (-13.6673, 5.1667) (-13.6643, 5.1651) (-13.6613, 5.1636) (-13.6584, 5.1622) (-13.6555, 5.1607) (-13.6527, 5.1593) (-13.6499, 5.1579) (-13.6472, 5.1566) (-13.6445, 5.1553) (-13.6419, 5.154) (-13.6393, 5.1528) (-13.6368, 5.1515) (-13.6343, 5.1504) (-13.6319, 5.1492) (-13.6296, 5.1481) (-13.6273, 5.147) (-13.625, 5.146) (-13.6228, 5.1449) (-13.6207, 5.1439) (-13.6186, 5.143) (-13.6166, 5.1421) (-13.6147, 5.1412) (-13.6128, 5.1403) (-13.6109, 5.1395) (-13.6091, 5.1387) (-13.6074, 5.1379) (-13.6057, 5.1372) (-13.6042, 5.1365) (-13.6026, 5.1358) (-13.6011, 5.1352) (-13.5997, 5.1346) (-13.5984, 5.134) (-13.5971, 5.1335) (-13.5959, 5.1329) (-13.5948, 5.1325) (-13.5937, 5.132) (-13.5927, 5.1316) (-13.5918, 5.1312) (-13.5909, 5.1309) (-13.5901, 5.1305) (-13.5894, 5.1303) (-13.5887, 5.13) (-13.5882, 5.1298) (-13.5877, 5.1296) (-13.5873, 5.1294) (-13.5871, 5.1293) (-13.587, 5.1293) (-13.5869, 5.1293) knots -1 -1 -1 -1 -1 -1 -0.99583333 -0.99166667 -0.9875 -0.98333333 -0.97916667 -0.975 -0.97083333 -0.96666667 -0.9625 -0.95833333 -0.95416667 -0.95 -0.94583333 -0.94166667 -0.9375 -0.93333333 -0.92916667 -0.925 -0.92083333 -0.91666667 -0.9125 -0.90833333 -0.90416667 -0.9 -0.89583333 -0.89166667 -0.8875 -0.88333333 -0.87916667 -0.875 -0.87083333 -0.86666667 -0.8625 -0.85833333 -0.85416667 -0.85 -0.84583333 -0.84166667 -0.8375 -0.83333333 -0.82916667 -0.825 -0.82083333 -0.81666667 -0.8125 -0.80833333 -0.80416667 -0.8 -0.79583333 -0.79166667 -0.7875 -0.78333333 -0.77916667 -0.775 -0.77083333 -0.76666667 -0.7625 -0.75833333 -0.75416667 -0.75 -0.74583333 -0.74166667 -0.7375 -0.73333333 -0.72916667 -0.725 -0.72083333 -0.71666667 -0.7125 -0.70833333 -0.70416667 -0.7 -0.69583333 -0.69166667 -0.6875 -0.68333333 -0.67916667 -0.675 -0.67083333 -0.66666667 -0.6625 -0.65833333 -0.65416667 -0.65 -0.64583333 -0.64166667 -0.6375 -0.63333333 -0.62916667 -0.625 -0.62083333 -0.61666667 -0.6125 -0.60833333 -0.60416667 -0.6 -0.59583333 -0.59166667 -0.5875 -0.58333333 -0.57916667 -0.575 -0.57083333 -0.56666667 -0.5625 -0.55833333 -0.55416667 -0.55 -0.54583333 -0.54166667 -0.5375 -0.53333333 -0.52916667 -0.525 -0.52083333 -0.51666667 -0.5125 -0.50833333 -0.50416667 -0.5 -0.49583333 -0.49166667 -0.4875 -0.48333333 -0.47916667 -0.475 -0.47083333 -0.46666667 -0.4625 -0.45833333 -0.45416667 -0.45 -0.44583333 -0.44166667 -0.4375 -0.43333333 -0.42916667 -0.425 -0.42083333 -0.41666667 -0.4125 -0.40833333 -0.40416667 -0.4 -0.39583333 -0.39166667 -0.3875 -0.38333333 -0.37916667 -0.375 -0.37083333 -0.36666667 -0.3625 -0.35833333 -0.35416667 -0.35 -0.34583333 -0.34166667 -0.3375 -0.33333333 -0.32916667 -0.325 -0.32083333 -0.31666667 -0.3125 -0.30833333 -0.30416667 -0.3 -0.29583333 -0.29166667 -0.2875 -0.28333333 -0.27916667 -0.275 -0.27083333 -0.26666667 -0.2625 -0.25833333 -0.25416667 -0.25 -0.24583333 -0.24166667 -0.2375 -0.23333333 -0.22916667 -0.225 -0.22083333 -0.21666667 -0.2125 -0.20833333 -0.20416667 -0.2 -0.19583333 -0.19166667 -0.1875 -0.18333333 -0.17916667 -0.175 -0.17083333 -0.16666667 -0.1625 -0.15833333 -0.15416667 -0.15 -0.14583333 -0.14166667 -0.1375 -0.13333333 -0.12916667 -0.125 -0.12083333 -0.11666667 -0.1125 -0.10833333 -0.10416667 -0.1 -0.09583333 -0.09166667 -0.0875 -0.08333333 -0.07916667 -0.075 -0.07083333 -0.06666667 -0.0625 -0.05833333 -0.05416667 -0.05 -0.04583333 -0.04166667 -0.0375 -0.03333333 -0.02916667 -0.025 -0.02083333 -0.01666667 -0.0125 -0.00833333 -0.00416667 0 0 0 0 0 0
  line L82 (-3.681, -14.0486) -> (-3.6808, -14.048)
  line L83 (-13.5869, 5.1293) -> (-13.5863, 5.129)